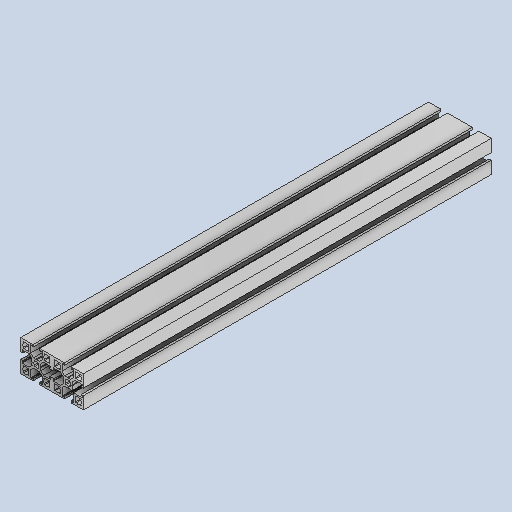
# Autodesk Inventor part: 3060 Aluminium Profile 390mm
Saved by Autodesk Inventor 2026.2 (Build 302298010, 298A)
## iProperties
Created: 2022-09-09
Part Number: 3060 Aluminium Profile 390mm
Material: Aluminum 6061-AHC
Document SubType Name: Modeling
Designer: chanh
Density: 2.7 g/cm^3
Appearance: Aluminum - Dark
Author: chanh
Autodesk Inventor part; units mm, degrees
ref_plane "RIGHT" through (0, 0, 0) normal (1, 0, 0) x (0, 1, 0)
ref_plane "TOP" through (0, 0, 0) normal (0, 1, 0) x (-1, 0, 0)
sketch "Sketch2" plane through (0, 0, 0) normal (0, 0, 1) x (1, 0, 0)
  circle A0 centre (0, 0) radius 2.5
  circle A1 centre (10, 10) radius 3
  line L0 (-4.25, -4.25) -> (4.25, -4.25)
  line L1 (4.25, -4.25) -> (4.25, 4.25)
  line L2 (4.25, 4.25) -> (-4.25, 4.25)
  line L3 (-4.25, 4.25) -> (-4.25, -4.25)
  line L4 (-4.25, -4.25) -> (4.25, 4.25) construction
  line L5 (4.25, -4.25) -> (-4.25, 4.25) construction
  line L6 (15, 5) -> (15, 15)
  line L7 (15, 15) -> (5, 15)
  line L8 (5, 5) -> (15, 15) construction
  line L9 (15, 5) -> (5, 15) construction
  line L10 (5, 15) -> (3.15, 15)
  line L11 (3.15, 15) -> (3.15, 13)
  line L12 (3.15, 13) -> (4.15, 13)
  line L13 (4.15, 13) -> (4.15, 13.7)
  line L14 (4.15, 13.7) -> (5.5, 13.7)
  line L15 (0, 0) -> (10, 10) construction
  line L16 (5.5, 15) -> (5.5, 5.5)
  line L17 (5.5, 5.5) -> (15, 5.5)
  line L18 (2.8358, 4.25) -> (5.5, 6.9142)
  line L19 (12.4042, 7.5958) -> (7.5958, 12.4042) construction
  line L20 (12.1213, 7.313) -> (7.313, 12.1213)
  line L21 (7.8787, 12.687) -> (12.687, 7.8787)
  arc A2 (12.1213, 7.313) -> (12.687, 7.8787) centre (12.4042, 7.5958) ccw
  arc A3 (7.8787, 12.687) -> (7.313, 12.1213) centre (7.5958, 12.4042) ccw
  line L22 (-0.4, 4.25) -> (0, 3.85)
  line L23 (0, 3.85) -> (0.4, 4.25)
  line L24 (0, 4.25) -> (0, -4.25) construction
  line L25 (7.5958, 7.5958) -> (12.4042, 12.4042) construction
  line L26 (7.8787, 7.313) -> (12.687, 12.1213)
  line L27 (12.1213, 12.687) -> (7.313, 7.8787)
  arc A4 (7.313, 7.8787) -> (7.8787, 7.313) centre (7.5958, 7.5958) ccw
  arc A5 (12.687, 12.1213) -> (12.1213, 12.687) centre (12.4042, 12.4042) ccw
  line L28 (15, 5) -> (15, 3.15)
  line L29 (15, 3.15) -> (13, 3.15)
  line L30 (13, 3.15) -> (13, 4.15)
  line L31 (13, 4.15) -> (13.7, 4.15)
  line L32 (13.7, 4.15) -> (13.7, 5.5)
  line L33 (4.25, 2.8358) -> (6.9142, 5.5)
  line L34 (-1.7678, -1.7678) -> (1.7678, 1.7678) construction
  line L35 (-1.4142, -2.1213) -> (2.1213, 1.4142)
  line L36 (1.4142, 2.1213) -> (-2.1213, -1.4142)
  arc A6 (-2.1213, -1.4142) -> (-1.4142, -2.1213) centre (-1.7678, -1.7678) ccw
  arc A7 (2.1213, 1.4142) -> (1.4142, 2.1213) centre (1.7678, 1.7678) ccw
  line L37 (1.7678, -1.7678) -> (-1.7678, 1.7678) construction
  line L38 (2.1213, -1.4142) -> (-1.4142, 2.1213)
  line L39 (-2.1213, 1.4142) -> (1.4142, -2.1213)
  arc A8 (1.4142, -2.1213) -> (2.1213, -1.4142) centre (1.7678, -1.7678) ccw
  arc A9 (-1.4142, 2.1213) -> (-2.1213, 1.4142) centre (-1.7678, 1.7678) ccw
  line L40 (-4.25, 0) -> (4.25, 0) construction
  circle A10 centre (10, -10) radius 3
  line L41 (15, -5) -> (15, -15)
  line L42 (15, -15) -> (5, -15)
  line L43 (5, -5) -> (15, -15) construction
  line L44 (15, -5) -> (5, -15) construction
  line L45 (5, -15) -> (3.15, -15)
  line L46 (3.15, -15) -> (3.15, -13)
  line L47 (3.15, -13) -> (4.15, -13)
  line L48 (4.15, -13) -> (4.15, -13.7)
  line L49 (4.15, -13.7) -> (5.5, -13.7)
  line L50 (0, 0) -> (10, -10) construction
  line L51 (5.5, -15) -> (5.5, -5.5)
  line L52 (5.5, -5.5) -> (15, -5.5)
  line L53 (2.8358, -4.25) -> (5.5, -6.9142)
  line L54 (12.4042, -7.5958) -> (7.5958, -12.4042) construction
  line L55 (12.1213, -7.313) -> (7.313, -12.1213)
  line L56 (7.8787, -12.687) -> (12.687, -7.8787)
  arc A11 (12.687, -7.8787) -> (12.1213, -7.313) centre (12.4042, -7.5958) ccw
  arc A12 (7.313, -12.1213) -> (7.8787, -12.687) centre (7.5958, -12.4042) ccw
  line L57 (7.5958, -7.5958) -> (12.4042, -12.4042) construction
  line L58 (7.8787, -7.313) -> (12.687, -12.1213)
  line L59 (12.1213, -12.687) -> (7.313, -7.8787)
  arc A13 (7.8787, -7.313) -> (7.313, -7.8787) centre (7.5958, -7.5958) ccw
  arc A14 (12.1213, -12.687) -> (12.687, -12.1213) centre (12.4042, -12.4042) ccw
  line L60 (13.7, -4.15) -> (13.7, -5.5)
  line L61 (15, -5) -> (15, -3.15)
  line L62 (15, -3.15) -> (13, -3.15)
  line L63 (13, -4.15) -> (13.7, -4.15)
  line L64 (13, -3.15) -> (13, -4.15)
  line L65 (4.25, -2.8358) -> (6.9142, -5.5)
  circle A15 centre (-10, 10) radius 3
  line L66 (-15, 5) -> (-15, 15)
  line L67 (-15, 15) -> (-5, 15)
  line L68 (-5, 5) -> (-15, 15) construction
  line L69 (-15, 5) -> (-5, 15) construction
  line L70 (-5, 15) -> (-3.15, 15)
  line L71 (-3.15, 15) -> (-3.15, 13)
  line L72 (-3.15, 13) -> (-4.15, 13)
  line L73 (-4.15, 13) -> (-4.15, 13.7)
  line L74 (-4.15, 13.7) -> (-5.5, 13.7)
  line L75 (0, 0) -> (-10, 10) construction
  line L76 (-5.5, 15) -> (-5.5, 5.5)
  line L77 (-5.5, 5.5) -> (-15, 5.5)
  line L78 (-2.8358, 4.25) -> (-5.5, 6.9142)
  line L79 (-12.4042, 7.5958) -> (-7.5958, 12.4042) construction
  line L80 (-12.1213, 7.313) -> (-7.313, 12.1213)
  line L81 (-7.8787, 12.687) -> (-12.687, 7.8787)
  arc A16 (-12.687, 7.8787) -> (-12.1213, 7.313) centre (-12.4042, 7.5958) ccw
  arc A17 (-7.313, 12.1213) -> (-7.8787, 12.687) centre (-7.5958, 12.4042) ccw
  line L82 (-7.5958, 7.5958) -> (-12.4042, 12.4042) construction
  line L83 (-7.8787, 7.313) -> (-12.687, 12.1213)
  line L84 (-12.1213, 12.687) -> (-7.313, 7.8787)
  arc A18 (-7.8787, 7.313) -> (-7.313, 7.8787) centre (-7.5958, 7.5958) ccw
  arc A19 (-12.1213, 12.687) -> (-12.687, 12.1213) centre (-12.4042, 12.4042) ccw
  line L85 (-13.7, 4.15) -> (-13.7, 5.5)
  line L86 (-15, 5) -> (-15, 3.15)
  line L87 (-15, 3.15) -> (-13, 3.15)
  line L88 (-13, 4.15) -> (-13.7, 4.15)
  line L89 (-13, 3.15) -> (-13, 4.15)
  line L90 (-4.25, 2.8358) -> (-6.9142, 5.5)
  arc A20 (-12.687, -12.1213) -> (-12.1213, -12.687) centre (-12.4042, -12.4042) ccw
  arc A21 (-7.8787, -12.687) -> (-7.313, -12.1213) centre (-7.5958, -12.4042) ccw
  arc A22 (-12.1213, -7.313) -> (-12.687, -7.8787) centre (-12.4042, -7.5958) ccw
  line L91 (-12.1213, -12.687) -> (-7.313, -7.8787)
  line L92 (-7.8787, -12.687) -> (-12.687, -7.8787)
  line L93 (-7.5958, -7.5958) -> (-12.4042, -12.4042) construction
  line L94 (-12.4042, -7.5958) -> (-7.5958, -12.4042) construction
  line L95 (-7.8787, -7.313) -> (-12.687, -12.1213)
  line L96 (-12.1213, -7.313) -> (-7.313, -12.1213)
  circle A23 centre (-10, -10) radius 3
  line L97 (-15, -15) -> (-5, -15)
  line L98 (-15, -5) -> (-15, -15)
  line L99 (-5.5, -15) -> (-5.5, -5.5)
  line L100 (-5.5, -5.5) -> (-15, -5.5)
  line L101 (-15, -5) -> (-5, -15) construction
  line L102 (-5, -5) -> (-15, -15) construction
  arc A24 (-7.313, -7.8787) -> (-7.8787, -7.313) centre (-7.5958, -7.5958) ccw
  line L103 (-5, -15) -> (-3.15, -15)
  line L104 (-3.15, -15) -> (-3.15, -13)
  line L105 (-4.15, -13) -> (-4.15, -13.7)
  line L106 (-4.15, -13.7) -> (-5.5, -13.7)
  line L107 (-3.15, -13) -> (-4.15, -13)
  line L108 (0, 0) -> (-10, -10) construction
  line L109 (-2.8358, -4.25) -> (-5.5, -6.9142)
  line L110 (-4.25, -2.8358) -> (-6.9142, -5.5)
  line L111 (-13.7, -4.15) -> (-13.7, -5.5)
  line L112 (-15, -5) -> (-15, -3.15)
  line L113 (-13, -3.15) -> (-13, -4.15)
  line L114 (-15, -3.15) -> (-13, -3.15)
  line L115 (-13, -4.15) -> (-13.7, -4.15)
  line L116 (-3.85, 0) -> (-4.25, 0.4)
  line L117 (-4.25, -0.4) -> (-3.85, 0)
  line L118 (0, -3.85) -> (-0.4, -4.25)
  line L119 (0.4, -4.25) -> (0, -3.85)
  line L120 (3.85, 0) -> (4.25, -0.4)
  line L121 (4.25, 0.4) -> (3.85, 0)
  circle A25 centre (30, 0) radius 2.5
  circle A26 centre (40, 10) radius 3
  line L122 (25.75, -4.25) -> (34.25, -4.25)
  line L123 (34.25, -4.25) -> (34.25, 4.25)
  line L124 (34.25, 4.25) -> (25.75, 4.25)
  line L125 (25.75, 4.25) -> (25.75, -4.25)
  line L126 (25.75, -4.25) -> (34.25, 4.25) construction
  line L127 (34.25, -4.25) -> (25.75, 4.25) construction
  line L128 (45, 5) -> (45, 15)
  line L129 (45, 15) -> (35, 15)
  line L130 (35, 5) -> (45, 15) construction
  line L131 (45, 5) -> (35, 15) construction
  line L132 (35, 15) -> (33.15, 15)
  line L133 (33.15, 15) -> (33.15, 13)
  line L134 (33.15, 13) -> (34.15, 13)
  line L135 (34.15, 13) -> (34.15, 13.7)
  line L136 (34.15, 13.7) -> (35.5, 13.7)
  line L137 (30, 0) -> (40, 10) construction
  line L138 (35.5, 15) -> (35.5, 5.5)
  line L139 (35.5, 5.5) -> (45, 5.5)
  line L140 (32.8358, 4.25) -> (35.5, 6.9142)
  line L141 (42.4042, 7.5958) -> (37.5958, 12.4042) construction
  line L142 (42.1213, 7.313) -> (37.313, 12.1213)
  line L143 (37.8787, 12.687) -> (42.687, 7.8787)
  arc A27 (42.1213, 7.313) -> (42.687, 7.8787) centre (42.4042, 7.5958) ccw
  arc A28 (37.8787, 12.687) -> (37.313, 12.1213) centre (37.5958, 12.4042) ccw
  line L144 (29.6, 4.25) -> (30, 3.85)
  line L145 (30, 3.85) -> (30.4, 4.25)
  line L146 (30, 4.25) -> (30, -4.25) construction
  line L147 (37.5958, 7.5958) -> (42.4042, 12.4042) construction
  line L148 (37.8787, 7.313) -> (42.687, 12.1213)
  line L149 (42.1213, 12.687) -> (37.313, 7.8787)
  arc A29 (37.313, 7.8787) -> (37.8787, 7.313) centre (37.5958, 7.5958) ccw
  arc A30 (42.687, 12.1213) -> (42.1213, 12.687) centre (42.4042, 12.4042) ccw
  line L150 (43.7, 4.15) -> (43.7, 5.5)
  line L151 (45, 5) -> (45, 3.15)
  line L152 (45, 3.15) -> (43, 3.15)
  line L153 (43, 4.15) -> (43.7, 4.15)
  line L154 (43, 3.15) -> (43, 4.15)
  line L155 (34.25, 2.8358) -> (36.9142, 5.5)
  line L156 (28.2322, -1.7678) -> (31.7678, 1.7678) construction
  line L157 (28.5858, -2.1213) -> (32.1213, 1.4142)
  line L158 (31.4142, 2.1213) -> (27.8787, -1.4142)
  arc A31 (27.8787, -1.4142) -> (28.5858, -2.1213) centre (28.2322, -1.7678) ccw
  arc A32 (32.1213, 1.4142) -> (31.4142, 2.1213) centre (31.7678, 1.7678) ccw
  line L159 (31.7678, -1.7678) -> (28.2322, 1.7678) construction
  line L160 (32.1213, -1.4142) -> (28.5858, 2.1213)
  line L161 (27.8787, 1.4142) -> (31.4142, -2.1213)
  arc A33 (31.4142, -2.1213) -> (32.1213, -1.4142) centre (31.7678, -1.7678) ccw
  arc A34 (28.5858, 2.1213) -> (27.8787, 1.4142) centre (28.2322, 1.7678) ccw
  line L162 (25.75, 0) -> (34.25, 0) construction
  arc A35 (42.1213, -12.687) -> (42.687, -12.1213) centre (42.4042, -12.4042) ccw
  arc A36 (37.313, -12.1213) -> (37.8787, -12.687) centre (37.5958, -12.4042) ccw
  arc A37 (42.687, -7.8787) -> (42.1213, -7.313) centre (42.4042, -7.5958) ccw
  line L163 (42.1213, -12.687) -> (37.313, -7.8787)
  line L164 (37.8787, -12.687) -> (42.687, -7.8787)
  line L165 (37.5958, -7.5958) -> (42.4042, -12.4042) construction
  line L166 (42.4042, -7.5958) -> (37.5958, -12.4042) construction
  line L167 (37.8787, -7.313) -> (42.687, -12.1213)
  line L168 (42.1213, -7.313) -> (37.313, -12.1213)
  circle A38 centre (40, -10) radius 3
  line L169 (45, -15) -> (35, -15)
  line L170 (45, -5) -> (45, -15)
  line L171 (35.5, -15) -> (35.5, -5.5)
  line L172 (35.5, -5.5) -> (45, -5.5)
  line L173 (45, -5) -> (35, -15) construction
  line L174 (35, -5) -> (45, -15) construction
  arc A39 (37.8787, -7.313) -> (37.313, -7.8787) centre (37.5958, -7.5958) ccw
  line L175 (35, -15) -> (33.15, -15)
  line L176 (33.15, -15) -> (33.15, -13)
  line L177 (34.15, -13) -> (34.15, -13.7)
  line L178 (34.15, -13.7) -> (35.5, -13.7)
  line L179 (33.15, -13) -> (34.15, -13)
  line L180 (30, 0) -> (40, -10) construction
  line L181 (32.8358, -4.25) -> (35.5, -6.9142)
  line L182 (34.25, -2.8358) -> (36.9142, -5.5)
  line L183 (43.7, -4.15) -> (43.7, -5.5)
  line L184 (45, -5) -> (45, -3.15)
  line L185 (43, -3.15) -> (43, -4.15)
  line L186 (45, -3.15) -> (43, -3.15)
  line L187 (43, -4.15) -> (43.7, -4.15)
  arc A40 (22.687, 12.1213) -> (22.1213, 12.687) centre (22.4042, 12.4042) ccw
  arc A41 (17.8787, 12.687) -> (17.313, 12.1213) centre (17.5958, 12.4042) ccw
  line L188 (17.8787, 12.687) -> (22.687, 7.8787)
  line L189 (22.1213, 12.687) -> (17.313, 7.8787)
  line L190 (22.4042, 7.5958) -> (17.5958, 12.4042) construction
  line L191 (17.5958, 7.5958) -> (22.4042, 12.4042) construction
  line L192 (22.1213, 7.313) -> (17.313, 12.1213)
  line L193 (17.8787, 7.313) -> (22.687, 12.1213)
  circle A42 centre (20, 10) radius 3
  line L194 (24.5, 15) -> (24.5, 5.5)
  line L195 (15, 15) -> (25, 15)
  line L196 (25, 5) -> (15, 15) construction
  line L197 (15, 5) -> (25, 15) construction
  line L198 (15, 5) -> (15, 15)
  line L199 (24.5, 5.5) -> (15, 5.5)
  arc A43 (17.313, 7.8787) -> (17.8787, 7.313) centre (17.5958, 7.5958) ccw
  line L200 (16.3, 4.15) -> (16.3, 5.5)
  line L201 (17, 4.15) -> (16.3, 4.15)
  line L202 (17, 3.15) -> (17, 4.15)
  line L203 (15, 5) -> (15, 3.15)
  line L204 (15, 3.15) -> (17, 3.15)
  line L205 (15, -5) -> (15, -3.15)
  arc A44 (22.1213, 7.313) -> (22.687, 7.8787) centre (22.4042, 7.5958) ccw
  line L206 (27.1642, -4.25) -> (24.5, -6.9142)
  line L207 (25.75, -2.8358) -> (23.0858, -5.5)
  line L208 (30, 0) -> (20, -10) construction
  arc A45 (22.687, -7.8787) -> (22.1213, -7.313) centre (22.4042, -7.5958) ccw
  line L209 (16.3, -4.15) -> (16.3, -5.5)
  line L210 (17, -4.15) -> (16.3, -4.15)
  line L211 (15, -3.15) -> (17, -3.15)
  line L212 (17, -3.15) -> (17, -4.15)
  line L213 (30, 0) -> (20, 10) construction
  line L214 (27.1642, 4.25) -> (24.5, 6.9142)
  line L215 (25.75, 2.8358) -> (23.0858, 5.5)
  arc A46 (17.8787, -7.313) -> (17.313, -7.8787) centre (17.5958, -7.5958) ccw
  line L216 (24.5, -5.5) -> (15, -5.5)
  arc A47 (17.313, -12.1213) -> (17.8787, -12.687) centre (17.5958, -12.4042) ccw
  line L217 (22.1213, -7.313) -> (17.313, -12.1213)
  line L218 (17.8787, -7.313) -> (22.687, -12.1213)
  line L219 (17.5958, -7.5958) -> (22.4042, -12.4042) construction
  line L220 (22.4042, -7.5958) -> (17.5958, -12.4042) construction
  line L221 (22.1213, -12.687) -> (17.313, -7.8787)
  line L222 (15, -5) -> (15, -15)
  line L223 (17.8787, -12.687) -> (22.687, -7.8787)
  circle A48 centre (20, -10) radius 3
  line L224 (25, -5) -> (15, -15) construction
  line L225 (15, -5) -> (25, -15) construction
  line L226 (24.5, -15) -> (24.5, -5.5)
  arc A49 (22.1213, -12.687) -> (22.687, -12.1213) centre (22.4042, -12.4042) ccw
  line L227 (15, -15) -> (25, -15)
  line L228 (25.85, -13.7) -> (24.5, -13.7)
  line L229 (25.85, 13.7) -> (24.5, 13.7)
  line L230 (25.85, 13) -> (25.85, 13.7)
  line L231 (26.85, 13) -> (25.85, 13)
  line L232 (26.85, 15) -> (26.85, 13)
  line L233 (25, 15) -> (26.85, 15)
  line L234 (25, -15) -> (26.85, -15)
  line L235 (26.85, -15) -> (26.85, -13)
  line L236 (26.85, -13) -> (25.85, -13)
  line L237 (25.85, -13) -> (25.85, -13.7)
  line L238 (26.15, 0) -> (25.75, 0.4)
  line L239 (25.75, -0.4) -> (26.15, 0)
  line L240 (30, -3.85) -> (29.6, -4.25)
  line L241 (30.4, -4.25) -> (30, -3.85)
  line L242 (33.85, 0) -> (34.25, -0.4)
  line L243 (34.25, 0.4) -> (33.85, 0)
  point P0 (-7.6148, -8.1805)
  point P1 (-7.6148, -11.8195)
  point P2 (-8.1805, -12.3852)
  point P3 (-11.8195, -12.3852)
  point P4 (-12.3852, -11.8195)
  point P5 (-12.3852, -8.1805)
  point P6 (-11.8195, -7.6148)
  point P7 (-8.1805, -7.6148)
  point P8 (-7.6148, 11.8195)
  point P9 (-7.6148, 8.1805)
  point P10 (-8.1805, 7.6148)
  point P11 (-11.8195, 7.6148)
  point P12 (-12.3852, 8.1805)
  point P13 (-12.3852, 11.8195)
  point P14 (-11.8195, 12.3852)
  point P15 (-8.1805, 12.3852)
  point P16 (11.8195, -12.3852)
  point P17 (8.1805, -12.3852)
  point P18 (7.6148, -11.8195)
  point P19 (7.6148, -8.1805)
  point P20 (8.1805, -7.6148)
  point P21 (11.8195, -7.6148)
  point P22 (12.3852, -8.1805)
  point P23 (12.3852, -11.8195)
  point P24 (-2.0856, -1.3785)
  point P25 (-2.0856, 1.3785)
  point P26 (-1.3785, 2.0856)
  point P27 (1.3785, 2.0856)
  point P28 (2.0856, 1.3785)
  point P29 (2.0856, -1.3785)
  point P30 (1.3785, -2.0856)
  point P31 (-1.3785, -2.0856)
  point P32 (11.8195, 7.6148)
  point P33 (8.1805, 7.6148)
  point P34 (7.6148, 8.1805)
  point P35 (7.6148, 11.8195)
  point P36 (8.1805, 12.3852)
  point P37 (11.8195, 12.3852)
  point P38 (12.3852, 11.8195)
  point P39 (12.3852, 8.1805)
  point P40 (0, 0)
  point P41 (41.8195, -12.3852)
  point P42 (38.1805, -12.3852)
  point P43 (37.6148, -11.8195)
  point P44 (37.6148, -8.1805)
  point P45 (38.1805, -7.6148)
  point P46 (41.8195, -7.6148)
  point P47 (42.3852, -8.1805)
  point P48 (42.3852, -11.8195)
  point P49 (18.1805, -7.6148)
  point P50 (21.8195, -7.6148)
  point P51 (22.3852, -8.1805)
  point P52 (22.3852, -11.8195)
  point P53 (21.8195, -12.3852)
  point P54 (18.1805, -12.3852)
  point P55 (17.6148, -11.8195)
  point P56 (17.6148, -8.1805)
  point P57 (27.9144, -1.3785)
  point P58 (27.9144, 1.3785)
  point P59 (28.6215, 2.0856)
  point P60 (31.3785, 2.0856)
  point P61 (32.0856, 1.3785)
  point P62 (32.0856, -1.3785)
  point P63 (31.3785, -2.0856)
  point P64 (28.6215, -2.0856)
  point P65 (41.8195, 7.6148)
  point P66 (38.1805, 7.6148)
  point P67 (37.6148, 8.1805)
  point P68 (37.6148, 11.8195)
  point P69 (38.1805, 12.3852)
  point P70 (41.8195, 12.3852)
  point P71 (42.3852, 11.8195)
  point P72 (42.3852, 8.1805)
  point P73 (22.3852, 11.8195)
  point P74 (22.3852, 8.1805)
  point P75 (21.8195, 7.6148)
  point P76 (18.1805, 7.6148)
  point P77 (17.6148, 8.1805)
  point P78 (17.6148, 11.8195)
  point P79 (18.1805, 12.3852)
  point P80 (21.8195, 12.3852)
  dimension "d15" = 5
  dimension "d16" = 6
  dimension "d17" = 10
  dimension "d18" = 10
  dimension "d19" = 8.5
  dimension "d21" = 3.15
  dimension "d22" = 1
  dimension "d23" = 2
  dimension "d24" = 1.3
  dimension "d25" = 5
  dimension "d26" = 4.5
  dimension "d27" = 1
  dimension "d28" = 0.8
  dimension "d29" = 3.4
  dimension "d30" = 0.8
  dimension "d31" = 0.8
  dimension "d32" = 3.4
  dimension "d33" = 1
  dimension "d34" = 1
  dimension "d37" = 360
  dimension "d43" = 5
  dimension "d44" = 6
  dimension "d45" = 10
  dimension "d46" = 10
  dimension "d47" = 8.5
  dimension "d48" = 3.15
  dimension "d49" = 1
  dimension "d50" = 2
  dimension "d51" = 1.3
  dimension "d52" = 5
  dimension "d53" = 4.5
  dimension "d54" = 1
  dimension "d55" = 0.8
  dimension "d56" = 3.4
  dimension "d57" = 0.8
  dimension "d58" = 0.8
  dimension "d59" = 3.4
  dimension "d60" = 1
  dimension "d61" = 1
  dimension "d62" = 360
  dimension "d63" = 21.5
  constraints: 528 end point, 224 symmetric about line, 84 point on circle, 76 point on line, 50 centre point, 34 midpoint, 32 tangent, 20 perpendicular, 14 parallel, 4 horizontal, 2 coincident, 2 collinear, 2 vertical, 1 horizontal alignment, 72 other
  measures "d15" diameter of A0
  measures "d16" diameter of A1
  measures "d17" horizontal distance of L15.end point (0, 0)
  measures "d18" horizontal distance of L15.end point (0, 0)
  measures "d19" distance of L2.end L1.end
  measures "d21" distance from line of L11 point (0, 0)
  measures "d22" distance between parallel lines of L13 L11
  measures "d23" distance between parallel lines of L12 L10
  measures "d24" distance between parallel lines of L10 L14
  measures "d25" horizontal distance of L6.end L15.end
  measures "d26" distance from line of L15.end L16
  measures "d27" distance between parallel lines of L8 L18
  measures "d28" distance between parallel lines of L21 L20
  measures "d29" distance of L15.end L19.end
  measures "d30" distance of L23.end L22.start
  measures "d31" diameter of A5
  measures "d32" distance of L25.end L15.end
  measures "d33" diameter of A7
  measures "d34" diameter of A9
  measures "d43" diameter of A25
  measures "d44" diameter of A26
  measures "d45" horizontal distance of L137.end point (30, 0)
  measures "d46" horizontal distance of L137.end point (30, 0)
  measures "d47" distance of L125.start L123.end
  measures "d48" distance from line of L133 point (30, 0)
  measures "d49" distance between parallel lines of L135 L133
  measures "d50" distance between parallel lines of L134 L132
  measures "d51" distance between parallel lines of L132 L136
  measures "d52" horizontal distance of L129.start L137.end
  measures "d53" distance from line of L137.end L138
  measures "d54" distance between parallel lines of L130 L140
  measures "d55" distance between parallel lines of L143 L142
  measures "d56" distance of L137.end L141.end
  measures "d57" distance of L145.end L144.start
  measures "d58" diameter of A30
  measures "d59" distance of L147.end L137.end
  measures "d60" diameter of A32
  measures "d61" diameter of A34
  measures "d63" distance between parallel lines of L125 L1
extrude "Extrusion2" add sketch "Sketch2" along normal blind 390 contours L3 L117 L116 L2 L22 L23 L1 L121 L120 L0 L119 L118 | L0 L109 L99 L100 L110 L3 | L99 L97 L98 L100 | L106 L105 L107 L104 L103 L97 L99 | L100 L98 L112 L114 L113 L115 L111 | L0 L1 L65 L52 L51 L53 | L90 L77 L76 L78 L2 L3 | L51 L52 L41 L42 | L77 L66 L67 L76 | L51 L42 L45 L46 L47 L48 L49 | L85 L88 L89 L87 L86 L66 L77 | L60 L63 L64 L62 L61 L41 L52 | L41 L216 L226 L227 | L76 L67 L70 L71 L72 L73 L74 | L1 L2 L18 L16 L17 L33 | L41 L61 L211 L212 L210 L209 L216 | L226 L228 L237 L236 L235 L234 L227 | L17 L16 L7 L6 | L17 L6 L28 L29 L30 L31 L32 | L207 L125 L122 L206 L226 L216 | L14 L13 L12 L11 L10 L7 L16 | L199 L200 L201 L202 L204 L28 L6 | L6 L195 L194 L199 | L125 L239 L238 L124 L144 L145 L123 L243 L242 L122 L241 L240 | L195 L233 L232 L231 L230 L229 L194 | L199 L194 L214 L124 L125 L215 | L171 L172 L170 L169 | L171 L169 L175 L176 L179 L177 L178 | L183 L187 L185 L186 L184 L170 L172 | L140 L138 L139 L155 L123 L124 | L138 L129 L128 L139 | L136 L135 L134 L133 L132 L129 L138 | L139 L128 L151 L152 L154 L153 L150
ref_plane "Work Plane2" through (0, 0, 195) normal (0, 0, -1) x (-1, 0, 0)
sketch "Sketch3" plane through (-15, 3.15, 0) normal (-1, 0, 0) x (0, 0, 1)
  line L0 (0, -3.15) -> (390, -3.15) projected
  line L1 (0, 311.85) -> (0, -98.15) projected
  line L2 (390, 311.85) -> (390, -98.15) projected
  line L3 (0, 11.85) -> (390, 11.85) projected
  line L4 (0, -18.15) -> (390, -18.15) projected
  line L5 (195, 11.85) -> (195, -18.15) construction
  line L6 (180, -3.15) -> (210, -3.15)
  point P0 (195, -3.15)
  dimension "d64" = 30
  constraints: 4 end point, 4 midpoint, 1 horizontal
  measures "d64" distance of L6.end L6.start
hole "Hole1" at (-15, 0, 180) at (-15, 0, 210) direction (1, 0, 0) diameter 6.2 end through all
body "Solid2"
